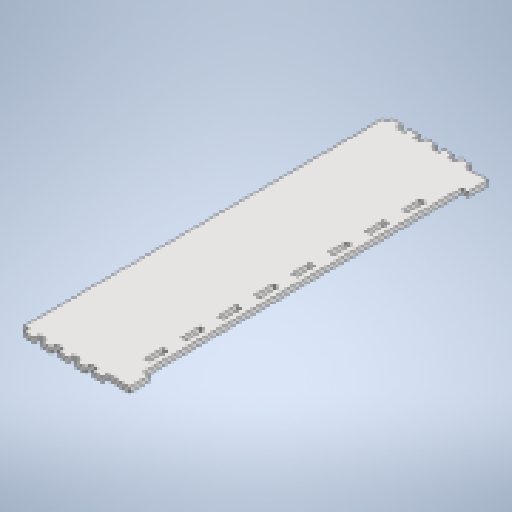
# Autodesk Inventor part: back
Saved by Autodesk Inventor 2025.3 (Build 293356000, 356)
## iProperties
Created: 2025-12-09
Part Number: back
Material: Generic
Document SubType Name: Modeling
Designer: hazem
Density: 1 g/cm^3
Appearance: Default
Author: hazem
Autodesk Inventor part; units mm, degrees
ref_plane "YZ Plane" through (0, 0, 0) normal (1, 0, 0) x (0, 1, 0)
ref_plane "XZ Plane" through (0, 0, 0) normal (0, 1, 0) x (-1, 0, 0)
ref_plane "XY Plane" through (0, 0, 0) normal (0, 0, 1) x (1, 0, 0)
sketch "Sketch1" plane through (0, 0, 0) normal (0, 1, 0) x (-1, 0, 0)
  line L0 (-71.6259, 7.6308) -> (8.4741, 7.6308)
  line L1 (8.4741, 7.6308) -> (8.4741, -292.3692)
  line L2 (8.4741, -292.3692) -> (-71.6259, -292.3692)
  line L3 (-71.6259, -292.3692) -> (-71.6259, 7.6308)
  point P0 (0, 0)
  constraints: 8 end point, 2 parallel, 1 horizontal, 1 perpendicular
extrude "Extrusion1" add sketch "Sketch1" along normal blind 4
sketch "Sketch2" plane through (0, 0, 0) normal (0, -1, 0) x (1, 0, 0)
  line L0 (-0.3741, 7.6308) -> (-18.4741, 7.6308) construction
  line L1 (-0.3741, 3.6308) -> (-0.3741, 7.6308) construction
  line L2 (7.6259, 7.6308) -> (7.6259, 3.6308) construction
  line L3 (13.6259, 3.6308) -> (7.6259, 3.6308) construction
  line L4 (13.6259, 3.6308) -> (13.6259, 7.6308) construction
  line L5 (21.6259, 7.6308) -> (21.6259, 3.6308) construction
  line L6 (27.6259, 3.6308) -> (21.6259, 3.6308) construction
  line L7 (27.6259, 3.6308) -> (27.6259, 7.6308) construction
  line L8 (35.6259, 7.6308) -> (35.6259, 3.6308) construction
  line L9 (41.6259, 3.6308) -> (35.6259, 3.6308) construction
  line L10 (41.6259, 3.6308) -> (41.6259, 7.6308) construction
  line L11 (49.6259, 7.6308) -> (49.6259, 3.6308) construction
  line L12 (55.6259, 3.6308) -> (49.6259, 3.6308) construction
  line L13 (55.6259, 3.6308) -> (55.6259, 7.6308) construction
  line L14 (63.6259, 7.6308) -> (63.6259, 3.6308) construction
  line L15 (71.6259, 3.6308) -> (63.6259, 3.6308) construction
  line L16 (67.6259, 3.6308) -> (67.6259, -7.3692) projected
  line L17 (67.6259, -7.3692) -> (71.6259, -7.3692) projected
  line L18 (71.6259, 3.6308) -> (71.6259, -7.3692) projected
  line L19 (67.6259, 3.6308) -> (71.6259, 3.6308) projected
  line L20 (67.6259, -22.3692) -> (67.6259, -37.3692) projected
  line L21 (67.6259, -37.3692) -> (71.6259, -37.3692) projected
  line L22 (71.6259, -22.3692) -> (71.6259, -37.3692) projected
  line L23 (67.6259, -22.3692) -> (71.6259, -22.3692) projected
  line L24 (67.6259, -52.3692) -> (67.6259, -67.3692) projected
  line L25 (67.6259, -67.3692) -> (71.6259, -67.3692) projected
  line L26 (71.6259, -52.3692) -> (71.6259, -67.3692) projected
  line L27 (67.6259, -52.3692) -> (71.6259, -52.3692) projected
  line L28 (67.6259, -82.3692) -> (67.6259, -97.3692) projected
  line L29 (67.6259, -97.3692) -> (71.6259, -97.3692) projected
  line L30 (71.6259, -82.3692) -> (71.6259, -97.3692) projected
  line L31 (67.6259, -82.3692) -> (71.6259, -82.3692) projected
  line L32 (67.6259, -112.3692) -> (67.6259, -127.3692) projected
  line L33 (67.6259, -127.3692) -> (71.6259, -127.3692) projected
  line L34 (71.6259, -112.3692) -> (71.6259, -127.3692) projected
  line L35 (67.6259, -112.3692) -> (71.6259, -112.3692) projected
  line L36 (67.6259, -142.3692) -> (67.6259, -157.3692) projected
  line L37 (67.6259, -157.3692) -> (71.6259, -157.3692) projected
  line L38 (71.6259, -142.3692) -> (71.6259, -157.3692) projected
  line L39 (67.6259, -142.3692) -> (71.6259, -142.3692) projected
  line L40 (67.6259, -172.3692) -> (67.6259, -187.3692) projected
  line L41 (67.6259, -187.3692) -> (71.6259, -187.3692) projected
  line L42 (71.6259, -172.3692) -> (71.6259, -187.3692) projected
  line L43 (67.6259, -172.3692) -> (71.6259, -172.3692) projected
  line L44 (67.6259, -202.3692) -> (67.6259, -217.3692) projected
  line L45 (67.6259, -217.3692) -> (71.6259, -217.3692) projected
  line L46 (71.6259, -202.3692) -> (71.6259, -217.3692) projected
  line L47 (67.6259, -202.3692) -> (71.6259, -202.3692) projected
  line L48 (67.6259, -232.3692) -> (67.6259, -247.3692) projected
  line L49 (67.6259, -247.3692) -> (71.6259, -247.3692) projected
  line L50 (71.6259, -232.3692) -> (71.6259, -247.3692) projected
  line L51 (67.6259, -232.3692) -> (71.6259, -232.3692) projected
  line L52 (67.6259, -262.3692) -> (67.6259, -277.3692) projected
  line L53 (67.6259, -277.3692) -> (71.6259, -277.3692) projected
  line L54 (71.6259, -262.3692) -> (71.6259, -277.3692) projected
  line L55 (67.6259, -262.3692) -> (71.6259, -262.3692) projected
  line L56 (71.6259, -288.3692) -> (63.5259, -288.3692) projected
  line L57 (63.5259, -288.3692) -> (63.5259, -292.3692) projected
  line L58 (55.5259, -292.3692) -> (55.5259, -288.3692) projected
  line L59 (55.5259, -288.3692) -> (49.5259, -288.3692) projected
  line L60 (49.5259, -288.3692) -> (49.5259, -292.3692) projected
  line L61 (41.5259, -288.3692) -> (35.5259, -288.3692) projected
  line L62 (41.5259, -292.3692) -> (41.5259, -288.3692) projected
  line L63 (35.5259, -288.3692) -> (35.5259, -292.3692) projected
  line L64 (27.5259, -288.3692) -> (21.5259, -288.3692) projected
  line L65 (27.5259, -292.3692) -> (27.5259, -288.3692) projected
  line L66 (21.5259, -288.3692) -> (21.5259, -292.3692) projected
  line L67 (13.5259, -288.3692) -> (7.5259, -288.3692) projected
  line L68 (13.5259, -292.3692) -> (13.5259, -288.3692) projected
  line L69 (7.5259, -288.3692) -> (7.5259, -292.3692) projected
  line L70 (-8.4741, -292.3692) -> (-8.4741, 7.6308) projected
  line L71 (-8.4741, -22.3692) -> (-8.4741, -37.3692) projected
  line L72 (-8.4741, -37.3692) -> (-4.4741, -37.3692) projected
  line L73 (-4.4741, -22.3692) -> (-4.4741, -37.3692) projected
  line L74 (-8.4741, -22.3692) -> (-4.4741, -22.3692) projected
  line L75 (-8.4741, -52.3692) -> (-8.4741, -67.3692) projected
  line L76 (-8.4741, -67.3692) -> (-4.4741, -67.3692) projected
  line L77 (-4.4741, -52.3692) -> (-4.4741, -67.3692) projected
  line L78 (-8.4741, -52.3692) -> (-4.4741, -52.3692) projected
  line L79 (-8.4741, -82.3692) -> (-8.4741, -97.3692) projected
  line L80 (-8.4741, -97.3692) -> (-4.4741, -97.3692) projected
  line L81 (-4.4741, -82.3692) -> (-4.4741, -97.3692) projected
  line L82 (-8.4741, -82.3692) -> (-4.4741, -82.3692) projected
  line L83 (-8.4741, -112.3692) -> (-8.4741, -127.3692) projected
  line L84 (-8.4741, -127.3692) -> (-4.4741, -127.3692) projected
  line L85 (-4.4741, -112.3692) -> (-4.4741, -127.3692) projected
  line L86 (-8.4741, -112.3692) -> (-4.4741, -112.3692) projected
  line L87 (-8.4741, -142.3692) -> (-8.4741, -157.3692) projected
  line L88 (-8.4741, -157.3692) -> (-4.4741, -157.3692) projected
  line L89 (-4.4741, -142.3692) -> (-4.4741, -157.3692) projected
  line L90 (-8.4741, -142.3692) -> (-4.4741, -142.3692) projected
  line L91 (-8.4741, -172.3692) -> (-8.4741, -187.3692) projected
  line L92 (-8.4741, -187.3692) -> (-4.4741, -187.3692) projected
  line L93 (-4.4741, -172.3692) -> (-4.4741, -187.3692) projected
  line L94 (-8.4741, -172.3692) -> (-4.4741, -172.3692) projected
  line L95 (-8.4741, -202.3692) -> (-8.4741, -217.3692) projected
  line L96 (-8.4741, -217.3692) -> (-4.4741, -217.3692) projected
  line L97 (-4.4741, -202.3692) -> (-4.4741, -217.3692) projected
  line L98 (-8.4741, -202.3692) -> (-4.4741, -202.3692) projected
  line L99 (-8.4741, -232.3692) -> (-8.4741, -247.3692) projected
  line L100 (-8.4741, -247.3692) -> (-4.4741, -247.3692) projected
  line L101 (-4.4741, -232.3692) -> (-4.4741, -247.3692) projected
  line L102 (-8.4741, -232.3692) -> (-4.4741, -232.3692) projected
  line L103 (71.6259, -37.1192) -> (67.6259, -37.1192)
  line L104 (67.6259, -22.6192) -> (71.6259, -22.6192)
  line L105 (67.6259, -52.6192) -> (71.6259, -52.6192)
  line L106 (71.6259, -67.1192) -> (67.6259, -67.1192)
  line L107 (67.6259, -82.6192) -> (71.6259, -82.6192)
  line L108 (71.6259, -97.1192) -> (67.6259, -97.1192)
  line L109 (67.6259, -112.6192) -> (71.6259, -112.6192)
  line L110 (71.6259, -127.1192) -> (67.6259, -127.1192)
  line L111 (67.6259, -142.6192) -> (71.6259, -142.6192)
  line L112 (71.6259, -157.1192) -> (67.6259, -157.1192)
  line L113 (67.6259, -172.6192) -> (71.6259, -172.6192)
  line L114 (71.6259, -187.1192) -> (67.6259, -187.1192)
  line L115 (67.6259, -202.6192) -> (71.6259, -202.6192)
  line L116 (71.6259, -217.1192) -> (67.6259, -217.1192)
  line L117 (67.6259, -232.6192) -> (71.6259, -232.6192)
  line L118 (71.6259, -247.1192) -> (67.6259, -247.1192)
  line L119 (67.6259, -262.6192) -> (71.6259, -262.6192)
  line L120 (71.6259, -277.1192) -> (67.6259, -277.1192)
  line L121 (-4.4741, -22.6192) -> (-8.4741, -22.6192)
  line L122 (-4.4741, -37.1192) -> (-8.4741, -37.1192)
  line L123 (-4.4741, -52.6192) -> (-8.4741, -52.6192)
  line L124 (-4.4741, -67.1192) -> (-8.4741, -67.1192)
  line L125 (-4.4741, -82.6192) -> (-8.4741, -82.6192)
  line L126 (-4.4741, -97.1192) -> (-8.4741, -97.1192)
  line L127 (-4.4741, -112.6192) -> (-8.4741, -112.6192)
  line L128 (-4.4741, -127.1192) -> (-8.4741, -127.1192)
  line L129 (-4.4741, -142.6192) -> (-8.4741, -142.6192)
  line L130 (-4.4741, -157.1192) -> (-8.4741, -157.1192)
  line L131 (-4.4741, -172.6192) -> (-8.4741, -172.6192)
  line L132 (-4.4741, -187.1192) -> (-8.4741, -187.1192)
  line L133 (-4.4741, -202.6192) -> (-8.4741, -202.6192)
  line L134 (-4.4741, -217.1192) -> (-8.4741, -217.1192)
  line L135 (-4.4741, -232.6192) -> (-8.4741, -232.6192)
  line L136 (-4.4741, -247.1192) -> (-8.4741, -247.1192)
  line L137 (7.8759, 7.6308) -> (7.8759, 3.6308)
  line L138 (13.3759, 3.6308) -> (13.3759, 7.6308)
  line L139 (21.8759, 7.6308) -> (21.8759, 3.6308)
  line L140 (27.3759, 3.6308) -> (27.3759, 7.6308)
  line L141 (35.8759, 7.6308) -> (35.8759, 3.6308)
  line L142 (41.3759, 3.6308) -> (41.3759, 7.6308)
  line L143 (49.8759, 7.6308) -> (49.8759, 3.6308)
  line L144 (55.3759, 3.6308) -> (55.3759, 7.6308)
  line L145 (7.7759, -292.3692) -> (7.7759, -288.3692)
  line L146 (13.2759, -288.3692) -> (13.2759, -292.3692)
  line L147 (21.7759, -292.3692) -> (21.7759, -288.3692)
  line L148 (27.2759, -288.3692) -> (27.2759, -292.3692)
  line L149 (35.7759, -292.3692) -> (35.7759, -288.3692)
  line L150 (41.2759, -288.3692) -> (41.2759, -292.3692)
  line L151 (49.7759, -292.3692) -> (49.7759, -288.3692)
  line L152 (55.2759, -288.3692) -> (55.2759, -292.3692)
  line L153 (13.6259, 3.6308) -> (7.6259, 3.6308) projected
  line L154 (27.6259, 3.6308) -> (21.6259, 3.6308) projected
  line L155 (41.6259, 3.6308) -> (35.6259, 3.6308) projected
  line L156 (55.6259, 3.6308) -> (49.6259, 3.6308) projected
  line L157 (71.6259, -292.3692) -> (-8.4741, -292.3692) projected
  line L158 (-0.3741, 3.6308) -> (-0.3741, 7.6308) projected
  line L159 (-8.4741, 7.6308) -> (71.6259, 7.6308) projected
  line L160 (71.6259, 7.6308) -> (71.6259, -292.3692) projected
  line L161 (63.6259, 7.6308) -> (63.6259, 3.6308) projected
  line L162 (71.6259, 3.6308) -> (63.6259, 3.6308) projected
  line L163 (-0.3741, 3.6308) -> (-18.4741, 3.6308) projected
  line L164 (-18.4741, 7.6308) -> (-18.4741, 3.6308) projected
  line L165 (-0.3741, 7.6308) -> (-18.4741, 7.6308) projected
  line L166 (-0.3741, 3.6308) -> (-0.3741, 7.6308) projected
  line L167 (-0.3741, 7.6308) -> (-18.4741, 7.6308) projected
  line L168 (-18.4741, 7.6308) -> (-18.4741, 3.6308) projected
  line L169 (-0.3741, 3.6308) -> (-18.4741, 3.6308) projected
  line L170 (-0.4741, -292.3692) -> (-0.4741, -288.3692) projected
  line L171 (-0.4741, -288.3692) -> (-18.4741, -288.3692) projected
  line L172 (-18.4741, -292.3692) -> (-18.4741, -288.3692) projected
  line L173 (-0.4741, -292.3692) -> (-18.4741, -292.3692) projected
  line L174 (18.1084, -192.1281) -> (2.6152, -192.1281)
  line L175 (2.6152, -192.1281) -> (2.6152, -222.247)
  line L176 (2.6152, -222.247) -> (18.1084, -222.247)
  line L177 (18.1084, -222.247) -> (18.1084, -192.1281)
  line L178 (-8.4741, -7.3692) -> (-4.4741, -7.3692)
  line L179 (-4.4741, -7.3692) -> (-4.4741, 7.6308)
  line L180 (-4.4741, 7.6308) -> (-8.4741, 7.6308)
  line L181 (-8.4741, 7.6308) -> (-8.4741, -7.3692)
  line L182 (-8.4741, -262.3692) -> (-4.4741, -262.3692)
  line L183 (-4.4741, -52.6192) -> (-4.4741, -288.3692)
  line L184 (-4.4741, -277.3692) -> (-8.4741, -277.3692)
  line L185 (-8.4741, -277.3692) -> (-8.4741, -262.3692)
  line L186 (-4.4741, -52.6192) -> (-4.4741, -7.3692)
  point P0 (0, 0)
  point P1 (-4.4741, -247.1192)
  point P2 (-4.4741, -232.6192)
  point P3 (-4.4741, -217.1192)
  point P4 (-4.4741, -202.6192)
  point P5 (-4.4741, -187.1192)
  point P6 (-4.4741, -172.6192)
  point P7 (-4.4741, -157.1192)
  point P8 (-4.4741, -142.6192)
  point P9 (-4.4741, -127.1192)
  point P10 (-4.4741, -112.6192)
  point P11 (-4.4741, -97.1192)
  point P12 (-4.4741, -82.6192)
  point P13 (-4.4741, -67.1192)
  point P14 (-4.4741, -52.6192)
  point P15 (-4.4741, 3.6308)
  point P16 (-8.4741, 3.6308)
  point P17 (-8.4741, -288.3692)
  dimension "d4" = 0.25
  dimension "d7" = 30
  dimension "d12" = 0.25
  dimension "d15" = 30
  dimension "d20" = 0.25
  dimension "d23" = 14
  dimension "d28" = 0.25
  dimension "d31" = 14
  dimension "d46" = 4
  dimension "d47" = 15
  dimension "d48" = 30
  dimension "d49" = 30
  constraints: 126 end point, 13 point on line, 6 horizontal, 6 parallel, 4 perpendicular, 3 vertical, 2 collinear, 150 other
  measures "d4" distance between parallel lines of L23 L104
  measures "d7" distance of L104.start L105.start
  measures "d12" distance between parallel lines of L103 L21
  measures "d15" distance of L123.start L121.start
  measures "d20" distance between parallel lines of L2 L137
  measures "d23" distance of L137.start L139.start
  measures "d28" distance between parallel lines of L69 L145
  measures "d31" distance of L145.start L147.start
  measures "d46" distance of L180.end L179.end
  measures "d47" distance of L179.end L178.end
  measures "d48" distance between parallel lines of L178 L72
  measures "d49" distance between parallel lines of L102 L182
extrude "Extrusion2" cut sketch "Sketch2" against normal through all contours L19 L18 L17 L16 | L162 L161 L159 L160 L19 | L22 L104 L20 L23 | L144 L156 L143 L159 | L22 L103 L20 L104 | L22 L21 L20 L103 | L142 L155 L141 L159 | L26 L105 L24 L27 | L140 L154 L139 L159 | L26 L106 L24 L105 | L26 L25 L24 L106 | L138 L153 L137 L159 | L30 L107 L28 L31 | L158 L163 L179 L159 | L30 L108 L28 L107 | L179 L163 L70 L159 | L30 L29 L28 L108 | L179 L178 L70 L163 | L70 L163 L164 L165 | L186 L74 L70 L178 | L34 L109 L32 L35 | L73 L121 L70 L74 | L34 L110 L32 L109 | L73 L122 L70 L121 | L34 L33 L32 L110 | L73 L72 L70 L122 | L186 L78 L70 L72 | L38 L111 L36 L39 | L77 L123 L70 L78 | L38 L112 L36 L111 | L77 L124 L70 L123 | L38 L37 L36 L112 | L77 L76 L70 L124 | L183 L82 L70 L76 | L42 L113 L40 L43 | L81 L125 L70 L82 | L42 L114 L40 L113 | L81 L126 L70 L125 | L42 L41 L40 L114 | L81 L80 L70 L126 | L183 L86 L70 L80 | L46 L115 L44 L47 | L85 L127 L70 L86 | L46 L116 L44 L115 | L85 L128 L70 L127 | L46 L45 L44 L116 | L85 L84 L70 L128 | L183 L90 L70 L84 | L50 L117 L48 L51 | L89 L129 L70 L90 | L50 L118 L48 L117 | L89 L130 L70 L129 | L50 L49 L48 L118 | L89 L88 L70 L130 | L183 L94 L70 L88 | L54 L119 L52 L55 | L93 L131 L70 L94 | L54 L120 L52 L119 | L93 L132 L70 L131 | L54 L53 L52 L120 | L93 L92 L70 L132 | L183 L98 L70 L92 | L160 L157 L57 L56 | L97 L133 L70 L98 | L97 L134 L70 L133 | L97 L96 L70 L134 | L157 L152 L59 L58 | L183 L102 L70 L96 | L157 L151 L59 L152 | L101 L135 L70 L102 | L157 L60 L59 L151 | L101 L136 L70 L135 | L101 L100 L70 L136 | L157 L150 L61 L62 | L183 L182 L70 L100 | L157 L149 L61 L150 | L183 L184 L70 L182 | L157 L63 L61 L149 | L183 L171 L70 L184 | L171 L170 L157 L70 | L157 L148 L64 L65 | L70 L173 L172 L171 | L157 L147 L64 L148 | L157 L66 L64 L147 | L69 L67 L145 L157 | L145 L67 L146 L157 | L157 L146 L67 L68
sketch "Sketch4" plane through (0, 4, 0) normal (0, 1, 0) x (1, 0, 0)
  line L0 (67.6259, 7.3692) -> (67.6259, -3.6308) projected
  line L1 (67.6259, -3.6308) -> (81.6259, -3.6308)
  line L2 (81.6259, -3.6308) -> (81.6259, 12.3692)
  line L3 (81.6259, 12.3692) -> (67.6259, 12.3692)
  line L4 (67.6259, 12.3692) -> (67.6259, -3.6308)
  line L5 (81.6259, -7.6308) -> (81.6259, -3.6308)
  line L6 (55.3759, -7.6308) -> (63.6259, -7.6308) projected
  line L7 (63.5259, 288.3692) -> (71.6259, 288.3692) projected
  line L8 (66.2844, 288.3692) -> (81.6259, 288.3692)
  line L9 (81.6259, 288.3692) -> (81.6259, 272.3692)
  line L10 (81.6259, 272.3692) -> (66.2844, 272.3692)
  line L11 (66.2844, 272.3692) -> (66.2844, 288.3692)
  line L12 (63.5259, 292.3692) -> (81.6259, 292.3692)
  line L13 (67.6259, 262.3692) -> (67.6259, 277.3692) projected
  line L14 (71.6259, 262.1619) -> (67.6259, 262.1619)
  line L15 (67.6259, 262.1619) -> (67.6259, 277.3692)
  line L16 (67.6259, 277.3692) -> (71.6259, 277.3692)
  line L17 (71.6259, 277.3692) -> (71.6259, 22.3692)
  line L18 (76.6259, 12.3692) -> (76.6259, 272.3692)
  line L19 (71.6259, 277.3692) -> (71.6259, 288.3692) projected
  line L20 (-0.4741, 292.3692) -> (-0.4741, 288.3692) projected
  line L21 (-0.4741, 288.3692) -> (-4.4741, 288.3692) projected
  line L22 (-4.4741, 288.3692) -> (-4.4741, -3.6308) projected
  line L23 (-4.4741, -3.6308) -> (-0.3741, -3.6308) projected
  line L24 (-0.3741, -3.6308) -> (-0.3741, -7.6308) projected
  line L25 (-0.3741, -7.6308) -> (7.8759, -7.6308) projected
  line L26 (7.8759, -7.6308) -> (7.8759, -3.6308) projected
  line L27 (7.8759, -3.6308) -> (13.3759, -3.6308) projected
  line L28 (13.3759, -3.6308) -> (13.3759, -7.6308) projected
  line L29 (13.3759, -7.6308) -> (21.8759, -7.6308) projected
  line L30 (21.8759, -7.6308) -> (21.8759, -3.6308) projected
  line L31 (21.8759, -3.6308) -> (27.3759, -3.6308) projected
  line L32 (27.3759, -3.6308) -> (27.3759, -7.6308) projected
  line L33 (27.3759, -7.6308) -> (35.8759, -7.6308) projected
  line L34 (35.8759, -7.6308) -> (35.8759, -3.6308) projected
  line L35 (35.8759, -3.6308) -> (41.3759, -3.6308) projected
  line L36 (41.3759, -3.6308) -> (41.3759, -7.6308) projected
  line L37 (41.3759, -7.6308) -> (49.8759, -7.6308) projected
  line L38 (49.8759, -7.6308) -> (49.8759, -3.6308) projected
  line L39 (49.8759, -3.6308) -> (55.3759, -3.6308) projected
  line L40 (55.3759, -3.6308) -> (55.3759, -7.6308) projected
  line L41 (55.3759, -7.6308) -> (63.6259, -7.6308) projected
  line L42 (63.6259, -7.6308) -> (63.6259, -3.6308) projected
  line L43 (63.6259, -3.6308) -> (67.6259, -3.6308) projected
  line L44 (67.6259, -3.6308) -> (67.6259, 7.3692) projected
  line L45 (67.6259, 7.3692) -> (71.6259, 7.3692) projected
  line L46 (71.6259, 7.3692) -> (71.6259, 22.3692) projected
  line L47 (71.6259, 22.3692) -> (67.6259, 22.3692) projected
  line L48 (67.6259, 22.3692) -> (67.6259, 37.3692) projected
  line L49 (67.6259, 37.3692) -> (71.6259, 37.3692) projected
  line L50 (71.6259, 37.3692) -> (71.6259, 52.3692) projected
  line L51 (71.6259, 52.3692) -> (67.6259, 52.3692) projected
  line L52 (67.6259, 52.3692) -> (67.6259, 67.3692) projected
  line L53 (67.6259, 67.3692) -> (71.6259, 67.3692) projected
  line L54 (71.6259, 67.3692) -> (71.6259, 82.3692) projected
  line L55 (71.6259, 82.3692) -> (67.6259, 82.3692) projected
  line L56 (67.6259, 82.3692) -> (67.6259, 97.3692) projected
  line L57 (67.6259, 97.3692) -> (71.6259, 97.3692) projected
  line L58 (71.6259, 97.3692) -> (71.6259, 112.3692) projected
  line L59 (71.6259, 112.3692) -> (67.6259, 112.3692) projected
  line L60 (67.6259, 112.3692) -> (67.6259, 127.3692) projected
  line L61 (67.6259, 127.3692) -> (71.6259, 127.3692) projected
  line L62 (71.6259, 127.3692) -> (71.6259, 142.3692) projected
  line L63 (71.6259, 142.3692) -> (67.6259, 142.3692) projected
  line L64 (67.6259, 142.3692) -> (67.6259, 157.3692) projected
  line L65 (67.6259, 157.3692) -> (71.6259, 157.3692) projected
  line L66 (71.6259, 157.3692) -> (71.6259, 172.3692) projected
  line L67 (71.6259, 172.3692) -> (67.6259, 172.3692) projected
  line L68 (67.6259, 172.3692) -> (67.6259, 187.3692) projected
  line L69 (67.6259, 187.3692) -> (71.6259, 187.3692) projected
  line L70 (71.6259, 187.3692) -> (71.6259, 202.3692) projected
  line L71 (71.6259, 202.3692) -> (67.6259, 202.3692) projected
  line L72 (67.6259, 202.3692) -> (67.6259, 217.3692) projected
  line L73 (67.6259, 217.3692) -> (71.6259, 217.3692) projected
  line L74 (71.6259, 217.3692) -> (71.6259, 232.3692) projected
  line L75 (71.6259, 232.3692) -> (67.6259, 232.3692) projected
  line L76 (67.6259, 232.3692) -> (67.6259, 247.3692) projected
  line L77 (67.6259, 247.3692) -> (71.6259, 247.3692) projected
  line L78 (71.6259, 247.3692) -> (71.6259, 262.3692) projected
  line L79 (71.6259, 262.3692) -> (67.6259, 262.3692) projected
  line L80 (67.6259, 262.3692) -> (67.6259, 277.3692) projected
  line L81 (67.6259, 277.3692) -> (71.6259, 277.3692) projected
  line L82 (71.6259, 277.3692) -> (71.6259, 288.3692) projected
  line L83 (71.6259, 288.3692) -> (63.5259, 288.3692) projected
  line L84 (63.5259, 288.3692) -> (63.5259, 292.3692) projected
  line L85 (63.5259, 292.3692) -> (55.5259, 292.3692) projected
  line L86 (55.5259, 292.3692) -> (55.5259, 288.3692) projected
  line L87 (55.5259, 288.3692) -> (49.5259, 288.3692) projected
  line L88 (49.5259, 288.3692) -> (49.5259, 292.3692) projected
  line L89 (49.5259, 292.3692) -> (41.5259, 292.3692) projected
  line L90 (41.5259, 292.3692) -> (41.5259, 288.3692) projected
  line L91 (41.5259, 288.3692) -> (35.5259, 288.3692) projected
  line L92 (35.5259, 288.3692) -> (35.5259, 292.3692) projected
  line L93 (35.5259, 292.3692) -> (27.5259, 292.3692) projected
  line L94 (27.5259, 292.3692) -> (27.5259, 288.3692) projected
  line L95 (27.5259, 288.3692) -> (21.5259, 288.3692) projected
  line L96 (21.5259, 288.3692) -> (21.5259, 292.3692) projected
  line L97 (21.5259, 292.3692) -> (13.5259, 292.3692) projected
  line L98 (13.5259, 292.3692) -> (13.5259, 288.3692) projected
  line L99 (13.5259, 288.3692) -> (7.5259, 288.3692) projected
  line L100 (7.5259, 288.3692) -> (7.5259, 292.3692) projected
  line L101 (7.5259, 292.3692) -> (-0.4741, 292.3692) projected
  point P0 (0, 0)
  point P1 (71.6259, 272.3692)
  point P2 (67.6259, 272.3692)
  point P3 (71.6259, 12.3692)
  dimension "d50" = 20
  dimension "d51" = 20
  dimension "d54" = 5
  constraints: 30 end point, 7 parallel, 5 point on line, 4 horizontal, 3 perpendicular, 2 collinear, 1 vertical, 4 other
  measures "d50" distance between parallel lines of L6 L3
  measures "d51" distance between parallel lines of L10 L12
  measures "d54" distance between parallel lines of L17 L18
extrude "Extrusion4" add sketch "Sketch4" against normal up to surface (4 mm away) contours L45 L46 L3 L2 L1 L0 | L4 L3 L46 L45 | L46 L17 L10 L18 L3 | L10 L17 L19 L8 L9 | L17 L79 L13 L10 | L10 L13 L16 L17 | L10 L11 L7 L19 L16 L13 | L17 L14 L15 L79
equation "\"d12\" = d4"
body "Solid1"
